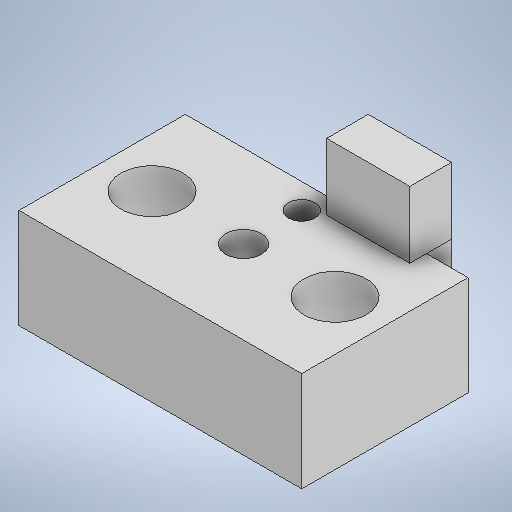
# Autodesk Inventor part: Taster_Schlitten_M8
Saved by Autodesk Inventor 2025 (Build 290162000, 162)
## iProperties
Created: 2026-07-09
Part Number: Taster_Schlitten_M8
Material: Generisch
Document SubType Name: Modeling
Designer: wavid
Mass: 58.2257 g
Surface Area: 163.883 cm^2
Volume: 58.2257 cm^3
Density: 1 g/cm^3
Appearance: Vorgabe
Author: wavid
Autodesk Inventor part; units mm, degrees
ref_plane "YZ Plane" through (0, 0, 0) normal (1, 0, 0) x (0, 1, 0)
sketch "Skizze1" plane through (0, 0, 0) normal (0, 0, 1) x (1, 0, 0)
  line L0 (-34, -20) -> (34, -20)
  line L1 (34, -20) -> (34, 20)
  line L2 (34, 20) -> (-34, 20)
  line L3 (-34, 20) -> (-34, -20)
  constraints: 8 end point, 2 parallel, 1 horizontal, 1 perpendicular
extrude "Extrusion1" add sketch "Skizze1" along normal blind 24
sketch "Skizze2" plane through (0, 0, 0) normal (0, 0, 1) x (1, 0, 0)
  line L0 (4, 20) -> (24, 20)
  line L1 (24, 20) -> (24, 26)
  line L2 (24, 26) -> (4, 26)
  line L3 (4, 26) -> (4, 20)
  constraints: 8 end point, 2 parallel, 1 horizontal, 1 perpendicular
extrude "Extrusion2" add sketch "Skizze2" along normal blind 24 separate body
ref_plane "Arbeitsebene1" through (0, 0, 24) normal (0, 0, 1) x (1, 0, 0)
sketch "Skizze3" plane through (0, 0, 24) normal (0, 0, 1) x (1, 0, 0)
  line L0 (4, 16) -> (24, 16)
  line L1 (24, 16) -> (24, 26)
  line L2 (24, 26) -> (4, 26)
  line L3 (4, 26) -> (4, 16)
  constraints: 8 end point, 2 parallel, 1 horizontal, 1 perpendicular
extrude "Extrusion3" add sketch "Skizze3" along normal blind 16 separate body
sketch "Skizze4" plane through (0, 0, 24) normal (0, 0, 1) x (1, 0, 0)
  circle A0 centre (-22, 0) radius 7.5
  constraints: 1 centre point
extrude "Extrusion4" cut sketch "Skizze4" against normal blind 24.2 bodies 1
sketch "Skizze5" plane through (0, 0, 24) normal (0, 0, 1) x (1, 0, 0)
  circle A0 centre (22, 0) radius 7.5
  constraints: 1 centre point
extrude "Extrusion5" cut sketch "Skizze5" against normal blind 24.2 bodies 1
sketch "Skizze6" plane through (0, 0, 24) normal (0, 0, 1) x (1, 0, 0)
  circle A0 centre (0, 0) radius 4.3
  constraints: 1 centre point
extrude "Extrusion6" cut sketch "Skizze6" against normal blind 24.2 bodies 1
sketch "Skizze7" plane through (0, 0, 24) normal (0, 0, 1) x (1, 0, 0)
  circle A0 centre (0, 14) radius 3.2
  constraints: 1 centre point
extrude "Extrusion7" cut sketch "Skizze7" against normal blind 24.2 bodies 1
sketch "Skizze8" plane through (0, 0, 0) normal (0, 0, 1) x (1, 0, 0)
  line L0 (-6.7, -7.8) -> (6.7, -7.8)
  line L1 (6.7, -7.8) -> (6.7, 7.8)
  line L2 (6.7, 7.8) -> (-6.7, 7.8)
  line L3 (-6.7, 7.8) -> (-6.7, -7.8)
  constraints: 8 end point, 2 parallel, 1 horizontal, 1 perpendicular
extrude "Extrusion8" cut sketch "Skizze8" along normal blind 7 bodies 1
sketch "Skizze9" plane through (0, 0, 0) normal (0, 0, 1) x (1, 0, 0)
  circle A0 centre (0, 14) radius 6.5
  constraints: 1 centre point
extrude "Extrusion9" cut sketch "Skizze9" along normal blind 14 bodies 1
sketch "Skizze10" plane through (0, 0, 0) normal (0, 0, 1) x (1, 0, 0)
  circle A0 centre (-9, 14) radius 1
  constraints: 1 centre point
extrude "Extrusion10" cut sketch "Skizze10" along normal blind 8 bodies 1
sketch "Skizze11" plane through (0, 0, 0) normal (0, 0, 1) x (1, 0, 0)
  circle A0 centre (9, 14) radius 1
  constraints: 1 centre point
extrude "Extrusion11" cut sketch "Skizze11" along normal blind 8 bodies 1
ref_plane "Arbeitsebene2" through (0, 16, 0) normal (0, 1, 0) x (-1, 0, 0)
sketch "Skizze12" plane through (0, 16, 0) normal (0, 1, 0) x (-1, 0, 0)
  circle A0 centre (9, 34) radius 1.2
  constraints: 1 centre point
extrude "Extrusion12" cut sketch "Skizze12" along normal blind 10.2 bodies 1
sketch "Skizze13" plane through (0, 16, 0) normal (0, 1, 0) x (-1, 0, 0)
  circle A0 centre (18.5, 34) radius 1.2
  constraints: 1 centre point
extrude "Extrusion13" cut sketch "Skizze13" along normal blind 10.2 bodies 1
